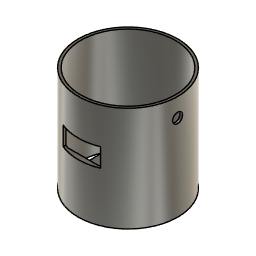
micro robot body (Autodesk Fusion 360 design; units mm, degrees)
Autodesk Fusion 360 part; units mm, degrees
note: some values were not read from the file. Set by a fixed rule: which sketch regions a step uses.
sketch "Sketch1" plane through (0, 0, 0) normal (0, 0, 1) x (1, 0, 0)
  circle A0 centre (0, 0) radius 40
  line L0 (0, 40) -> (0, -40) construction
  circle A1 centre (0, 0) radius 43
  line L1 (-26, 14.5) -> (-26, -14.5)
  line L2 (-40.4815, -14.5) -> (-26, -14.5)
  line L3 (-26, 14.5) -> (-40.4815, 14.5)
  line L4 (40, 0) -> (-40, 0) construction
  line L5 (26, 14.5) -> (40.4815, 14.5)
  line L6 (26, 14.5) -> (26, -14.5)
  line L7 (40.4815, -14.5) -> (26, -14.5)
  circle A2 centre (15, -9) radius 1.1
  circle A3 centre (15, 9) radius 1.1
  circle A4 centre (-15, -9) radius 1.1
  circle A5 centre (-15, 9) radius 1.1
  line L8 (-26, 14.5) -> (26, 14.5)
  line L9 (26, -14.5) -> (-26, -14.5)
  line L10 (17.5, -35.9687) -> (-17.5, -35.9687)
  dimension "d1" = 80
  dimension "d39" = 3
  dimension "d40" = 29
  dimension "d41" = 14
  dimension "d49" = 2.2
  dimension "d50" = 9
  dimension "d51" = 15
  dimension "d52" = 11
  dimension "d69" = 35
  constraint coincident A0.centre A1.centre
  constraint coincident A0 L0.start
  constraint coincident A0 L0.end
  constraint vertical L0
  constraint coincident A0.centre L0
  constraint vertical L1
  constraint coincident A1 L2.start
  constraint perpendicular L1 L2
  constraint coincident A1 L3.end
  constraint perpendicular L1 L3
  constraint coincident A0 L4.start
  constraint coincident A0 L4.end
  constraint horizontal L4
  constraint coincident A0.centre L4
  constraint symmetric L2 L3 L4
  constraint symmetric L0 L1.start L5.start
  constraint symmetric L0 L1.end L6.end
  constraint symmetric L0 L2.start L7.start
  constraint symmetric L0 L3.end L5.end
  constraint symmetric L4 A2 A3
  constraint symmetric L0 A2 A4
  constraint symmetric L0 A3 A5
  constraint coincident A0 L10.start
  constraint coincident A0 L10.end
  constraint perpendicular L0 L10
  measures "d1" diameter of A0
  measures "d40" distance of L2 L3
  measures "d41" distance of L1 L4.end
  measures "d49" diameter of A2
  measures "d50" distance of L4 A2.centre
  measures "d51" distance of L0 A2.centre
  measures "d52" distance of L1 A5.centre
  measures "d69" distance of L10.start L10.end
extrude "Extrude1" add sketch "Sketch1" along normal blind 4 contours A0 L10 | A0 L2 L7 L9 L10 | A0 L3 L5 L8 | L1 L6 L8 L9
sketch "Sketch3" plane through (0, 0, 4) normal (0, 0, 1) x (-1, 0, 0)
  circle A0 centre (0, 0) radius 38
  circle A1 centre (0, 0) radius 40
  line L0 (37.2794, -14.5) -> (26, -14.5)
  line L1 (26, -14.5) -> (26, 14.5)
  line L2 (26, 14.5) -> (37.2794, 14.5)
  line L3 (-26, 14.5) -> (-26, -14.5)
  line L4 (-26, -14.5) -> (-37.2794, -14.5)
  line L5 (-37.2794, 14.5) -> (-26, 14.5)
  circle A2 centre (-15, 9) radius 1.1
  circle A3 centre (15, -9) radius 1.1
  circle A4 centre (-15, -9) radius 1.1
  circle A5 centre (15, 9) radius 1.1
  arc A6 (-37.2794, -14.5) -> (37.2794, -14.5) centre (0, 0) ccw
  arc A7 (37.2794, 14.5) -> (-37.2794, 14.5) centre (0, 0) ccw
  dimension "d20" = 76
  dimension "d21" = 80
  constraint coincident A0.centre A1.centre
  constraint concentric A0 A1
  measures "d20" diameter of A0
  measures "d21" diameter of A1
extrude "Extrude7" add sketch "Sketch3" along normal blind 80 and the other way blind 4 contours A0 A1 L0 L2 | A0 A1 L2 L5 A7 | A0 A1 L0 L4 A6 | A0 A1 L4 L5
extrude "Extrude12" add sketch "Sketch1" along normal blind 9 contours L1 L6 L8 L9
sketch "Sketch7" plane through (0, 0, 0) normal (0, 1, 0) x (1, 0, 0)
  line L0 (-15, -55) -> (15, -55)
  line L1 (15, -55) -> (15, -40)
  line L2 (15, -40) -> (-15, -40)
  line L3 (-15, -40) -> (-15, -55)
  line L4 (0, 0) -> (0, -80) construction
  line L5 (15, -40) -> (-15, -40)
  line L6 (-15, -40) -> (-15, -37)
  line L7 (-15, -37) -> (15, -37)
  line L8 (15, -37) -> (15, -40)
  dimension "d63" = 30
  dimension "d64" = 15
  dimension "d65" = 80
  dimension "d68" = 3
  constraint horizontal L0
  constraint vertical L1
  constraint horizontal L2
  constraint vertical L3
  constraint coincident L4.start origin
  constraint vertical L4
  constraint midpoint L2 L4
  constraint horizontal L5
  constraint vertical L6
  constraint horizontal L7
  constraint vertical L8
  constraint collinear L3 L6
  measures "d63" distance of L0.start L0.end
  measures "d64" distance of L0.start L2.end
  measures "d65" distance of L4.start L4.end
  measures "d68" distance of L2.end L6.end
extrude "Extrude14" cut sketch "Sketch7" against normal blind 60 contours L0 L1 L2 L3 L5
extrude "Extrude15" add sketch "Sketch1" along normal blind 40 contours A0 L10
sketch "Sketch8" plane through (0, 0, 0) normal (1, 0, 0) x (0, 1, 0)
  circle A0 centre (0, 69) radius 4
  line L0 (40, 84) -> (-40, 84)
  dimension "d72" = 8
  dimension "d73" = 15
  measures "d72" diameter of A0
  measures "d73" distance of A0.centre L0
extrude "Extrude16" cut sketch "Sketch8" along normal blind 100
